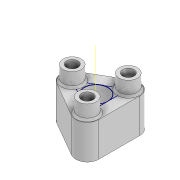
# Autodesk Inventor part: 9 rotor 2.0
Saved by Autodesk Inventor 2020 (Build 240168000, 168)
## iProperties
Created: 2020-05-08
Part Number: 9 rotor 2.0
Material: Generic
Document SubType Name: Modeling
Designer: mrbeh
Density: 1 g/cm^3
Appearance: Default
Author: mrbeh
Autodesk Inventor part; units mm, degrees
ref_plane "YZ Plane" through (0, 0, 0) normal (1, 0, 0) x (0, 1, 0)
ref_plane "XZ Plane" through (0, 0, 0) normal (0, 1, 0) x (-1, 0, 0)
ref_plane "XY Plane" through (0, 0, 0) normal (0, 0, 1) x (1, 0, 0)
sketch "Sketch1" plane through (0, 0, 0) normal (0, 1, 0) x (-1, 0, 0)
  line L0 (0, 0) -> (9.2925, -5.365)
  line L1 (0, 0) -> (10.73, 0) construction
  line L2 (9.2925, -5.365) -> (0, -10.73)
  line L3 (0, -10.73) -> (0, 0)
  dimension "d0" = 10.73
  dimension "d1" = 30
  dimension "d2" = 10.73
  dimension "d3" = 60
  constraints: 8 end point, 1 equal length, 1 horizontal
  measures "d0" distance of L0.start L0.end
  measures "d1" angle of L0 L1
  measures "d2" distance of L0.end L2.end
  measures "d3" angle of L0 L2
extrude "Extrusion1" add sketch "Sketch1" along normal blind 9
sketch "Sketch2" plane through (0, 9, 0) normal (0, 1, 0) x (1, 0, 0)
  line L0 (0, 0) -> (0, 10.73) projected
  circle A0 centre (0, 0) radius 2.3813
  dimension "d6" = 4.7625
  constraints: 1 centre point, 1 coincident
  measures "d6" diameter of A0
extrude "Extrusion2" add sketch "Sketch2" along normal blind 3.7
sketch "Sketch8" plane through (0, 9, 0) normal (0, 1, 0) x (1, 0, 0)
  line L0 (0, 10.73) -> (-9.2925, 5.365) projected
  line L1 (-9.2925, 5.365) -> (0, 10.73)
  line L2 (0, 0) -> (0, 10.73) projected
  line L3 (0, 10.73) -> (0, 0)
  line L4 (0, 0) -> (-9.2925, 5.365)
  circle A0 centre (-3.0975, 5.365) radius 3.0975
  constraints: 6 end point, 3 tangent, 2 collinear, 1 centre point
pattern_circular "Circular Pattern3" count 3 over 360 about axis through (-3.0975, 9, -5.365) along (0, 1, 0) of "Extrusion2"
thicken "Thicken2" operation add thickness 3 both sides no extend neighbours no toward (1, 0, 0) faces at (0, 3, -6.3596) (-5.5076, 3, -7.5502) (-5.5076, 3, -3.1798)
fillet "Fillet2" radius 3 3 edges at (3, 4.5, 5.1962) (3, 4.5, -15.9262) (-15.2925, 4.5, -5.365)
chamfer "Chamfer3" distance 0.5 angle 45 3 edges at (1.1906, 9, -8.6678) (-2.3813, 9, 0) (-8.1018, 9, -7.4272)
sketch "Sketch11" plane through (0, 9, 0) normal (0, 1, 0) x (1, 0, 0)
  circle A0 centre (-3.0975, 5.365) radius 3.225
  point P0 (0, 0)
  dimension "d39" = 6.45
  constraints: 1 centre point
  measures "d39" diameter of A0
extrude "Extrusion5" cut sketch "Sketch11" against normal blind 10
sketch "Sketch12" plane through (0, 12.7, 0) normal (0, 1, 0) x (1, 0, 0)
  circle A0 centre (0, 0) radius 1.5
  dimension "d42" = 3
  constraints: 1 centre point, 1 coincident
  measures "d42" diameter of A0
extrude "Extrusion6" cut sketch "Sketch12" against normal blind 20
pattern_circular "Circular Pattern4" count 3 over 360 about axis through (-3.0975, 9, -5.365) along (0, 1, 0) of "Extrusion6"
body "Solid1"
